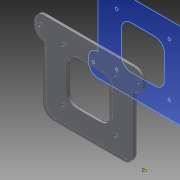
# Autodesk Inventor part: Bolt Cradel
Saved by Autodesk Inventor 2015 (Build 190159000, 159)
## iProperties
Created: 2014-11-13
Part Number: Bolt Cradel
Material: Generic
Document SubType Name: Modeling
Designer: karl
Density: 1 g/cm^3
Appearance: Default
Author: karl
Autodesk Inventor part; units mm, degrees
ref_plane "YZ Plane" through (0, 0, 0) normal (1, 0, 0) x (0, 1, 0)
ref_plane "XZ Plane" through (0, 0, 0) normal (0, 1, 0) x (-1, 0, 0)
ref_plane "XY Plane" through (0, 0, 0) normal (0, 0, 1) x (1, 0, 0)
sketch "Sketch1" plane through (0, 0, 0) normal (0, 1, 0) x (-1, 0, 0)
  line L0 (-47, -45) -> (47, -45)
  line L1 (47, -45) -> (47, 45)
  line L2 (47, 45) -> (-47, 45)
  line L3 (-47, 45) -> (-47, -45)
  line L4 (-47, -45) -> (47, 45) construction
  line L5 (47, -45) -> (-47, 45) construction
  point P0 (0, 0)
  dimension "d0" = 94
  dimension "d1" = 90
  constraints: 12 end point, 2 midpoint, 2 parallel, 1 horizontal, 1 perpendicular
  measures "d0" distance of L2.end L1.end
  measures "d1" distance of L1.end L0.end
extrude "Extrusion1" add sketch "Sketch1" along normal blind 3
sketch "Sketch2" plane through (0, 0, 0) normal (0, -1, 0) x (1, 0, 0)
  line L0 (-47, 45) -> (-57, 45)
  line L1 (-57, 45) -> (-57, 21)
  line L2 (-57, 21) -> (-47, 21)
  line L3 (-47, 21) -> (-47, 45)
  line L4 (47, -45) -> (-47, -45) projected
  point P0 (0, 0)
  dimension "d4" = 10
  dimension "d5" = 66
  constraints: 8 end point, 2 parallel, 1 horizontal, 1 perpendicular
  measures "d4" distance of L2.end L1.end
  measures "d5" distance between parallel lines of L2 L4
extrude "Extrusion2" add sketch "Sketch2" against normal blind 3
sketch "Sketch3" plane through (0, 0, 0) normal (0, -1, 0) x (1, 0, 0)
  line L0 (-30, 30) -> (30, 30) construction
  line L1 (30, 30) -> (30, -30) construction
  line L2 (30, -30) -> (-30, -30) construction
  line L3 (-30, -30) -> (-30, 30) construction
  line L4 (-30, 30) -> (30, -30) construction
  line L5 (30, 30) -> (-30, -30) construction
  circle A0 centre (-27.5, -27.5) radius 1.5
  circle A1 centre (27.5, -27.5) radius 1.5
  circle A2 centre (27.5, 27.5) radius 1.5
  circle A3 centre (-27.5, 27.5) radius 1.5
  point P0 (0, 0)
  dimension "d8" = 60
  dimension "d9" = 60
  dimension "d10" = 3
  dimension "d11" = 27.5
  dimension "d14" = 360
  constraints: 12 end point, 4 centre point, 2 midpoint, 2 parallel, 1 horizontal, 1 perpendicular, 1 point on line, 9 other
  measures "d8" distance of L1.end L2.end
  measures "d9" distance of L0.end L1.end
  measures "d10" diameter of A0
  measures "d11" horizontal distance of A0.centre point (0, 0)
extrude "Extrusion3" cut sketch "Sketch3" against normal blind 3
sketch "Sketch4" plane through (0, 0, 0) normal (0, -1, 0) x (1, 0, 0)
  line L0 (22.5, 22.5) -> (-22.5, 22.5)
  line L1 (-22.5, 22.5) -> (-22.5, -22.5)
  line L2 (-22.5, -22.5) -> (22.5, -22.5)
  line L3 (22.5, -22.5) -> (22.5, 22.5)
  line L4 (22.5, 22.5) -> (-22.5, -22.5) construction
  line L5 (-22.5, 22.5) -> (22.5, -22.5) construction
  point P0 (0, 0)
  dimension "d18" = 45
  dimension "d19" = 45
  constraints: 12 end point, 2 midpoint, 2 parallel, 1 horizontal, 1 perpendicular
  measures "d18" distance of L2.end L1.end
  measures "d19" distance of L1.end L0.end
extrude "Extrusion4" cut sketch "Sketch4" against normal blind 3
fillet "Fillet1" radius 10 3 edges at (-57, 1.5, 21) (-57, 1.5, 45) (-47, 1.5, -45)
mirror "Mirror1" about plane through (0, 0, 0) normal (1, 0, 0) of "Extrusion2", "Fillet1"
fillet "Fillet2" radius 10 4 edges at (-22.5, 1.5, -22.5) (22.5, 1.5, -22.5) (22.5, 1.5, 22.5) (-22.5, 1.5, 22.5)
sketch "Sketch5" plane through (0, 0, 0) normal (0, -1, 0) x (1, 0, 0)
  circle A0 centre (52, 33) radius 1.5
  line L0 (57, 35) -> (57, 31) projected
  point P0 (0, 0)
  point P1 (57, 33)
  dimension "d24" = 3
  dimension "d25" = 5
  constraints: 1 centre point, 1 horizontal alignment, 1 midpoint
  measures "d24" diameter of A0
  measures "d25" distance from line of L0 A0.centre
extrude "Extrusion5" cut sketch "Sketch5" against normal blind 3
mirror "Mirror2" about plane through (0, 0, 0) normal (1, 0, 0) of "Extrusion5"
body "Solid1"
